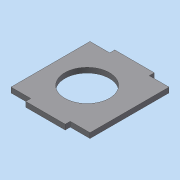
# Autodesk Inventor part: Part3
Saved by Autodesk Inventor 2016 SP1 (Build 200210100, 210)
## iProperties
Created: 2016-03-20
Part Number: Part3
Material: Generic
Document SubType Name: Modeling
Designer: Mohamed A.
Density: 1 g/cm^3
Appearance: Default
Author: Mohamed A.
Autodesk Inventor part; units mm, degrees
ref_plane "YZ Plane" through (0, 0, 0) normal (1, 0, 0) x (0, 1, 0)
ref_plane "XZ Plane" through (0, 0, 0) normal (0, 1, 0) x (-1, 0, 0)
ref_plane "XY Plane" through (0, 0, 0) normal (0, 0, 1) x (1, 0, 0)
sketch "Sketch1" plane through (0, 0, 0) normal (0, 0, 1) x (1, 0, 0)
  circle A0 centre (-1.6325, 0) radius 5.15 construction
  circle A1 centre (-1.6325, 0) radius 13.25 projected
  line L0 (10.9595, -23.5) -> (10.9595, 23.5) construction
  line L1 (-21.7072, 23.5) -> (-21.7072, -23.5) construction
  line L2 (11.8175, -23.5) -> (11.8175, -26.5)
  line L3 (11.8175, -26.5) -> (4.3175, -26.5)
  line L4 (-11.6825, -26.5) -> (-11.6825, -23.5)
  circle A2 centre (-1.6325, 0) radius 13.25 construction
  line L5 (-5.8325, -4.2) -> (-5.8325, 4.2) construction
  line L6 (-5.8325, 4.2) -> (12.0675, 4.2) construction
  line L7 (12.0675, 4.2) -> (12.0675, -4.2) construction
  line L8 (12.0675, -4.2) -> (-5.8325, -4.2) construction
  circle A3 centre (-17.9325, 18) radius 2.75 construction
  circle A4 centre (18.0675, 18) radius 2.75 construction
  circle A5 centre (-17.9325, -18) radius 2.75 construction
  circle A6 centre (18.0675, -18) radius 2.75 construction
  circle A7 centre (10.0175, 10.5) radius 2 construction
  circle A8 centre (-2.4825, 10.5) radius 2 construction
  circle A9 centre (-2.4825, -10.5) radius 2 construction
  circle A10 centre (10.0175, -10.5) radius 2 construction
  line L9 (-23.4325, 23.5) -> (-23.4325, -23.5) projected
  line L10 (-23.4325, -23.5) -> (-11.6825, -23.5)
  line L11 (23.5675, -23.5) -> (23.5675, 23.5) projected
  line L12 (23.5675, 23.5) -> (-23.4325, 23.5) construction
  line L13 (4.3175, -26.5) -> (4.3175, -23.5)
  line L14 (1.5675, -23.5) -> (1.5675, -21.5)
  line L15 (1.5675, -21.5) -> (2.7175, -21.5)
  line L16 (2.7175, -19.1) -> (2.7175, -21.5)
  line L17 (2.7175, -19.1) -> (1.5675, -19.1)
  line L18 (1.5675, -19.1) -> (1.5675, -18.5)
  line L19 (1.5675, -18.5) -> (-1.4325, -18.5)
  line L20 (-1.4325, -18.5) -> (-1.4325, -19.1)
  line L21 (-1.4325, -19.1) -> (-2.5825, -19.1)
  line L22 (-2.5825, -19.1) -> (-2.5825, -21.5)
  line L23 (-2.5825, -21.5) -> (-1.4325, -21.5)
  line L24 (-1.4325, -23.5) -> (-1.4325, -21.5)
  line L25 (-4.1825, -23.5) -> (-4.1825, -26.5)
  line L26 (0.0675, -17.369) -> (0.0675, -28.5133) construction
  line L27 (-4.1825, -26.5) -> (-11.6825, -26.5)
  line L28 (4.3175, -26.5) -> (-4.1825, -26.5) construction
  line L29 (1.5675, -23.5) -> (4.3175, -23.5)
  line L30 (-1.4325, -23.5) -> (-4.1825, -23.5)
  line L31 (-4.1825, -23.5) -> (-1.4325, -23.5)
  line L32 (-32.8325, 0) -> (32.9675, 0) construction
  line L33 (11.8175, -23.5) -> (23.5675, -23.5)
  line L34 (1.5675, -23.5) -> (4.3175, -23.5)
  line L35 (11.8175, 23.5) -> (11.8175, 26.5)
  line L36 (11.8175, 26.5) -> (4.3175, 26.5)
  line L37 (-11.6825, 26.5) -> (-11.6825, 23.5)
  line L38 (-23.4325, 23.5) -> (-11.6825, 23.5)
  line L39 (4.3175, 26.5) -> (4.3175, 23.5)
  line L40 (1.5675, 23.5) -> (1.5675, 21.5)
  line L41 (1.5675, 21.5) -> (2.7175, 21.5)
  line L42 (2.7175, 19.1) -> (2.7175, 21.5)
  line L43 (2.7175, 19.1) -> (1.5675, 19.1)
  line L44 (1.5675, 19.1) -> (1.5675, 18.5)
  line L45 (1.5675, 18.5) -> (-1.4325, 18.5)
  line L46 (-1.4325, 18.5) -> (-1.4325, 19.1)
  line L47 (-1.4325, 19.1) -> (-2.5825, 19.1)
  line L48 (-2.5825, 19.1) -> (-2.5825, 21.5)
  line L49 (-2.5825, 21.5) -> (-1.4325, 21.5)
  line L50 (-1.4325, 23.5) -> (-1.4325, 21.5)
  line L51 (-4.1825, 23.5) -> (-4.1825, 26.5)
  line L52 (-4.1825, 26.5) -> (-11.6825, 26.5)
  line L53 (1.5675, 23.5) -> (4.3175, 23.5)
  line L54 (-4.1825, 23.5) -> (-1.4325, 23.5)
  line L55 (11.8175, 23.5) -> (23.5675, 23.5)
  point P0 (0, 0)
  dimension "d11" = 47
  dimension "d12" = 11.75
  dimension "d15" = 11.75
  dimension "d16" = 3
  dimension "d18" = 3
  dimension "d19" = 5.3
  dimension "d20" = 2.4
  dimension "d21" = 5
  dimension "d22" = 8
  dimension "d23" = 7.5
  constraints: 90 end point, 26 point on line, 23 perpendicular, 20 symmetric about line, 8 collinear, 1 vertical, 4 other
  measures "d11" distance between parallel lines of L9 L11
  measures "d12" distance between parallel lines of L2 L11
  measures "d15" distance between parallel lines of L9 L4
  measures "d16" distance between parallel lines of L10 L3
  measures "d18" distance between parallel lines of L24 L14
  measures "d19" distance between parallel lines of L22 L16
  measures "d20" distance between parallel lines of L15 L17
  measures "d21" distance between parallel lines of L3 L15
  measures "d22" distance between parallel lines of L3 L19
  measures "d23" distance between parallel lines of L13 L2
extrude "Extrusion1" add sketch "Sketch1" along normal blind 3 contours A1 | L2 L3 L13 L29 L14 L15 L16 L17 L18 L19 L20 L21 L22 L23 L24 L30 L25 L27 L4 L10 L9 L38 L37 L52 L51 L54 L50 L49 L48 L47 L46 L45 L44 L43 L42 L41 L40 L53 L39 L36 L35 L55 L11 L33
equation "\"d12\" = 0.25 * d11"
equation "\"d15\" = d12"
body "Solid1"
